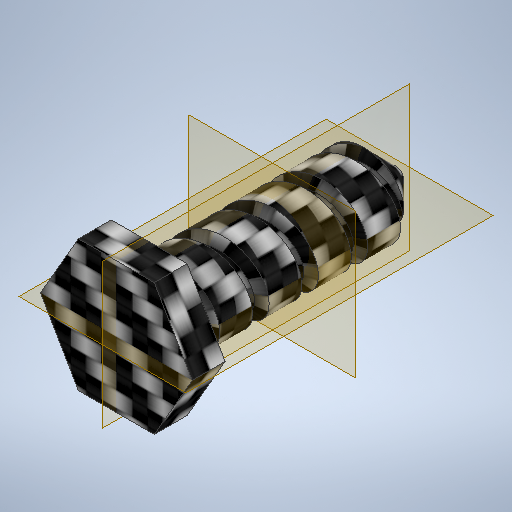
# Autodesk Inventor part: Peça_0003_001
Saved by Autodesk Inventor 2025.2 (Build 292293000, 293)
## iProperties
Created: 2025-03-25
Part Number: Peça_0003_001
Material: Ouro
Document SubType Name: Modeling
Designer: lucas
Density: 19.3 g/cm^3
Appearance: Fibra de carbono
Author: lucas
Autodesk Inventor part; units mm, degrees
sketch "Esboço1" plane through (0, 0, 0) normal (0, 0, 1) x (1, 0, 0)
  circle A0 centre (0, 0) radius 2.5
  dimension "d0" = 5
  constraints: 1 centre point, 1 coincident
  measures "d0" diameter of A0
extrude "Extrusão1" add sketch "Esboço1" along normal mid plane 15
sketch "Esboço2" plane through (0, 0, 0) normal (1, 0, 0) x (0, 1, 0)
  line L0 (2.5, -8.5) -> (1.634, -8) construction
  line L1 (1.634, -8) -> (2.5, -7.5) construction
  line L2 (2.5, -7.5) -> (2.5, -8.5)
  line L3 (-2.5, -7.5) -> (2.5, -7.5) construction
  arc A0 (1.934, -7.8268) -> (1.934, -8.1732) centre (2.034, -8) ccw
  line L4 (2.5, -7.5) -> (1.934, -7.8268)
  line L5 (1.934, -8.1732) -> (2.5, -8.5)
  point P0 (0, 0)
  point P1 (2.2113, -8)
  dimension "d6" = 1
  dimension "d7" = 0.2
  constraints: 10 end point, 2 collinear, 2 point on circle, 2 point on line, 2 tangent, 1 centre point, 1 vertical, 7 other
  measures "d6" distance of L1.end L0.start
  measures "d7" radius of A0
coil "Espiral1" sketch "Esboço2" operation cut axis through (0, 0, -10) along (0, 0, 1) pitch 3 turns 11.666667 hand right
chamfer "Chanfro1" distance 2 angle 45 2 edges at (1.7678, 1.7678, -7.5) (0.647, -2.4148, -7.5)
sketch "Esboço5" plane through (0, 0, 7.5) normal (0, 0, 1) x (1, 0, 0)
  line L0 (2.3094, 4) -> (4.6188, 0)
  line L1 (4.6188, 0) -> (2.3094, -4)
  line L2 (2.3094, -4) -> (-2.3094, -4)
  line L3 (-2.3094, -4) -> (-4.6188, 0)
  line L4 (-4.6188, 0) -> (-2.3094, 4)
  line L5 (-2.3094, 4) -> (2.3094, 4)
  point P0 (0, 0)
  point P1 (0, 0)
  dimension "d20" = 4
  constraints: 12 end point, 1 coincident, 1 horizontal, 13 other
  measures "d20" distance from line of point (0, 0) L5
extrude "Extrusão2" add sketch "Esboço5" along normal blind 2
